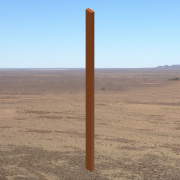
# Autodesk Inventor part: Pole_EdgeSupportUpright
Saved by Autodesk Inventor 2013 SP2 (Build 170200200, 200)
## iProperties
Created: 2013-09-03
Part Number: Pole_EdgeSupportUpright
Material: Wood (Cherry)
Document SubType Name: Modeling
Designer: Dave
Mass: 3355.25 g
Surface Area: 5099.99 cm^2
Volume: 6710.5 cm^3
Density: 0.5 g/cm^3
Author: Dave
Autodesk Inventor part; units mm, degrees
ref_plane "YZ Plane" through (0, 0, 0) normal (1, 0, 0) x (0, 1, 0)
ref_plane "XZ Plane" through (0, 0, 0) normal (0, 1, 0) x (-1, 0, 0)
ref_plane "XY Plane" through (0, 0, 0) normal (0, 0, 1) x (1, 0, 0)
sketch "Sketch1" plane through (0, 0, 0) normal (0, 1, 0) x (-1, 0, 0)
  line L0 (0, 0) -> (88.9, 0)
  line L1 (88.9, 0) -> (88.9, 38.1)
  line L2 (88.9, 38.1) -> (0, 38.1)
  line L3 (0, 38.1) -> (0, 0)
  dimension "d0" = 88.9
  dimension "d1" = 38.1
  constraints: 8 end point, 2 parallel, 1 horizontal, 1 perpendicular
  measures "d0" distance of L0.start L0.end
  measures "d1" distance of L2.end L0.start
extrude "Extrusion1" add sketch "Sketch1" along normal blind 1981.2
sketch "Sketch3" plane through (-88.9, 0, 38.1) normal (0, 0, 1) x (1, 0, 0)
  line L0 (0, 0) -> (88.9, 0) projected
  line L1 (0, 0) -> (0, 1981.2) projected
  circle A0 centre (25.4, 101.6) radius 5.7238
  circle A1 centre (63.5, 101.6) radius 5.7238
  circle A2 centre (25.4, 609.6) radius 5.7238
  circle A3 centre (63.5, 609.6) radius 5.7238
  dimension "d28" = 101.6
  dimension "d29" = 25.4
  dimension "d32" = 38.1
  dimension "d35" = 508
  constraints: 4 centre point, 1 horizontal, 1 vertical, 6 other
  measures "d28" distance from line of L0 A0.centre
  measures "d29" distance from line of A0.centre L1
  measures "d32" distance of A0.centre A1.centre
  measures "d35" distance of A0.centre A2.centre
hole "Hole2" at (-63.5, 609.6, 38.1) at (-25.4, 609.6, 38.1) at (-63.5, 101.6, 38.1) at (-25.4, 101.6, 38.1) direction (0, 0, -1) diameter 6.35 end through all
body "Solid1"
